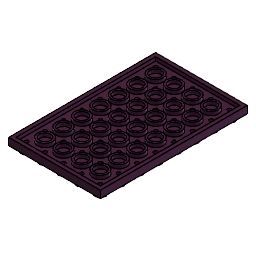
Parametric design Lego (Autodesk Fusion 360 design; units mm, degrees)
Autodesk Fusion 360 part; units mm, degrees
note: some values were not read from the file. Set by a fixed rule: which face or edge a step refers to.
sketch "Sketch1" plane through (0, 0, 0) normal (0, 1, 0) x (1, 0, 0) in component "Lego"
  line L0 (19.9, -31.9) -> (-19.9, -31.9)
  line L1 (-19.9, -31.9) -> (-19.9, 31.9)
  line L2 (-19.9, 31.9) -> (19.9, 31.9)
  line L3 (19.9, 31.9) -> (19.9, -31.9)
  line L4 (19.9, -31.9) -> (-19.9, 31.9) construction
  line L5 (-19.9, -31.9) -> (19.9, 31.9) construction
  dimension "d6" = 63.8
  dimension "d7" = 39.8
  constraint horizontal L0
  constraint perpendicular L0 L1
  constraint parallel L0 L2
  constraint parallel L1 L3
  constraint coincident L4 origin
  constraint coincident L5 origin
  measures "d6" distance of L0.start L2.end
  measures "d7" distance of L1.end L2.end
extrude "Extrude1" add sketch "Sketch1" along normal blind 3.2 in component "Lego"
sketch "Sketch2" plane through (0, 3.2, 0) normal (0, 1, 0) x (-1, 0, 0) in component "Lego"
  line L0 (-19.9, -31.9) -> (19.9, -31.9)
  line L1 (19.9, -31.9) -> (19.9, 31.9)
  line L2 (19.9, 31.9) -> (-19.9, 31.9)
  line L3 (-19.9, 31.9) -> (-19.9, -31.9)
  circle A0 centre (16, -28) radius 2.4
  dimension "d10" = 4.8
  dimension "d11" = 3.9
  dimension "d12" = 3.9
  measures "d10" diameter of A0
  measures "d11" distance of L0 A0.centre
  measures "d12" distance of L1 A0.centre
extrude "Extrude2" add sketch "Sketch2" along normal blind 1.8 contours A0 in component "Lego"
pattern_linear "R-Pattern1" count 8 spacing 8 along (0, 0, 1) count 5 spacing 8 along (1, 0, 0) of "Extrude2" in component "Lego"
shell "Shell1" thickness 1.6 removed faces 1 at (-6.6333, 0, -10.6333) in component "Lego"
sketch "Sketch3" plane through (0, 0, 0) normal (0, 1, 0) x (1, 0, 0) in component "Lego"
  circle A0 centre (-12, -24) radius 2.4
  circle A1 centre (-12, -24) radius 3.25
  point P0 (-19.9, -31.9)
  point P1 (-19.9, 31.9)
  dimension "d20" = 4.8
  dimension "d21" = 6.5
  dimension "d22" = 7.9
  dimension "d23" = 7.9
  constraint concentric A0 A1
  measures "d20" diameter of A0
  measures "d21" diameter of A1
  measures "d22" vertical distance of A0.centre P0
  measures "d23" horizontal distance of A0.centre P1
extrude "Extrude3" add sketch "Sketch3" along normal up to surface (3.2 mm away) in component "Lego"
pattern_linear "R-Pattern2" count 4 spacing 8 along (1, 0, 0) count 7 spacing 8 along (0, 0, -1) of "Extrude3" in component "Lego"
move_body "Move1" bodies 1 to x (1, 0, 0) y (0, -1, 0) z (0, 0, -1) at (0, 19.2, 8) in component "Lego"
component "Lego" placed x (1, 0, 0) y (0, 1, 0) z (0, 0, 1) at (0, 0, 0)
equation "LENGTH = 5"
equation "WIDTH = 8"
equation "HEIGHT = LOW"
equation "HIGH = 3 * LOW"
equation "LOW = 3.2 mm"
equation "d6 = ( WIDTH * 8 mm ) - 0.2 mm"
equation "d7 = ( LENGTH * 8 mm ) - 0.2 mm"
equation "d8 = HEIGHT"
equation "d15 = WIDTH"
equation "d16 = LENGTH"
equation "d26 = LENGTH - 1"
equation "d27 = WIDTH - 1"
